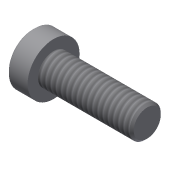
# Autodesk Inventor part: Bolt3RH
Saved by Autodesk Inventor 2022.5 (Build 265521000, 521)
## iProperties
Created: 2010-08-06
Part Number: Bolt3RH
Document SubType Name: Modeling
Designer: nguyenducthang
Density: 1 g/cm^3
Mass: 0.102158 g
Surface Area: 1.46803 cm^2
Volume: 0.102158 cm^3
Material: Generic
Appearance: Default
Author: nguyenducthang
Autodesk Inventor part; units mm, degrees
ref_plane "YZ Plane" through (0, 0, 0) normal (1, 0, 0) x (0, 1, 0)
ref_plane "XZ Plane" through (0, 0, 0) normal (0, 1, 0) x (-1, 0, 0)
ref_plane "XY Plane" through (0, 0, 0) normal (0, 0, 1) x (1, 0, 0)
sketch "Sketch15" plane through (0, 0, 0) normal (0, 0, 1) x (1, 0, 0)
  line L0 (0, 0) -> (0, 2.5)
  line L1 (0, 2.5) -> (2, 2.5)
  line L2 (3, 4.4) -> (3, 4.4)
  line L3 (2, 1.5) -> (11, 1.5)
  line L4 (11, 0) -> (0, 0)
  line L5 (11, 0) -> (7.2, 0)
  line L6 (2, 1.5) -> (2, 2.5)
  line L7 (11, 1.5) -> (11, 0)
  dimension "d84" = 1.5
  dimension "d87" = 2.5
  dimension "d116" = 2
  dimension "d117" = 9
  constraints: 16 end point, 4 parallel, 2 perpendicular, 1 vertical, 1 other
  measures "d84" distance between parallel lines of L3 L4
  measures "d87" distance between parallel lines of L1 L4
  measures "d116" distance between parallel lines of L0 L6
  measures "d117" distance of L3.start L3.end
revolve "Revolution1" add sketch "Sketch15" angle 360 about axis through (11, 0, 0) along (-1, 0, 0)
chamfer "Chamfer5" distance 0.2 angle 45 1 edges at (11, -1.5, 0)
thread "Thread8" size "M3x0.5" class "6g" standard "ANSI Metric M Profile" full length
sketch "Sketch20" plane through (0, 0, 0) normal (-1, 0, 0) x (0, 0, 1)
  line L0 (-1.25, 0.7217) -> (0, 1.4434)
  line L1 (0, 1.4434) -> (1.25, 0.7217)
  line L2 (1.25, 0.7217) -> (1.25, -0.7217)
  line L3 (1.25, -0.7217) -> (0, -1.4434)
  line L4 (0, -1.4434) -> (-1.25, -0.7217)
  line L5 (-1.25, -0.7217) -> (-1.25, 0.7217)
  point P0 (0, 0)
  point P1 (0, 0)
  dimension "d143" = 2.5
  constraints: 12 end point, 1 coincident, 13 other
  measures "d143" distance between parallel lines of L2 L5
extrude "Extrusion19" cut sketch "Sketch20" against normal blind 1.5
chamfer "Chamfer6" distance 0.2 angle 45 1 edges at (0, -2.5, 0)
body "Solid1"
